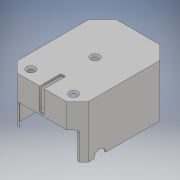
# Autodesk Inventor part: Kozhuh_Lock_Left
Saved by Autodesk Inventor 2017 (Build 210142000, 142)
## iProperties
Part Number: Kozhuh_Lock_Left
Material: Типовые
Document SubType Name: Modeling
Designer: yulia_000
Density: 1 g/cm^3
Appearance: По умолчанию
Author: yulia_000
## iProperties of the stored document Kozhuh_Lock_Right_3DПЕЧАТЬ.ipt
Part Number: Kozhuh_Lock_Right_3DПЕЧАТЬ
Material: Типовые
Document SubType Name: Modeling
Designer: Тетяна
Density: 1 g/cm^3
Appearance: По умолчанию
Author: Тетяна
Autodesk Inventor part; units mm, degrees
ref_plane "YZ Plane" through (0, 0, 0) normal (1, 0, 0) x (0, 1, 0)
ref_plane "XZ Plane" through (0, 0, 0) normal (0, 1, 0) x (-1, 0, 0)
ref_plane "XY Plane" through (0, 0, 0) normal (0, 0, 1) x (1, 0, 0)
sketch "Эскиз1" plane through (0, 0, 0) normal (0, 1, 0) x (-1, 0, 0)
  line L0 (11, 0) -> (47.6, 0)
  line L1 (58.6, -11) -> (58.6, -71.5)
  line L2 (50.1, -80) -> (8.5, -80)
  line L3 (0, -71.5) -> (0, -11)
  line L4 (58.6, -11) -> (47.6, 0)
  line L5 (58.6, -71.5) -> (50.1, -80)
  line L6 (8.5, -80) -> (0, -71.5)
  line L7 (0, -11) -> (11, 0)
  line L8 (59.8, -71.9971) -> (50.5971, -81.2)
  line L9 (50.5971, -81.2) -> (8.0029, -81.2)
  line L10 (8.0029, -81.2) -> (-1.2, -71.9971)
  line L11 (-1.2, -71.9971) -> (-1.2, -10.5029)
  line L12 (-1.2, -10.5029) -> (10.5029, 1.2)
  line L13 (10.5029, 1.2) -> (48.0971, 1.2)
  line L14 (48.0971, 1.2) -> (59.8, -10.5029)
  line L15 (59.8, -10.5029) -> (59.8, -71.9971)
  line L16 (31.3, -63) -> (27.3, -63)
  line L17 (27.3, -63) -> (27.3, -80)
  line L18 (27.3, -80) -> (31.3, -80)
  line L19 (31.3, -80) -> (31.3, -63)
  line L20 (31.3, -63) -> (27.3, -80) construction
  line L21 (27.3, -63) -> (31.3, -80) construction
  point P0 (0, 0)
  point P1 (58.6, -80)
  point P2 (58.6, 0)
  point P3 (0, -80)
  point P4 (29.3, -71.5)
  point P5 (29.3, -80)
  dimension "d8" = 58.6
  dimension "d9" = 80
  dimension "d10" = 11
  dimension "d11" = 11
  dimension "d12" = 8.5
  dimension "d13" = 8.5
  dimension "d14" = 8.5
  dimension "d15" = 8.5
  dimension "d16" = 11
  dimension "d17" = 11
  dimension "d18" = 1.2
  dimension "d51" = 4
  dimension "d52" = 17
  constraints: 44 end point, 8 point on line, 6 parallel, 4 midpoint, 3 perpendicular, 2 horizontal, 7 other
  measures "d8" distance of point (58.6, -80) point (0, -80)
  measures "d9" distance of point (58.6, 0) point (58.6, -80)
  measures "d10" distance of L1.start point (58.6, 0)
  measures "d11" distance of L0.end point (58.6, 0)
  measures "d12" distance of L1.end point (58.6, -80)
  measures "d13" distance of L2.start point (58.6, -80)
  measures "d14" distance of L2.end point (0, -80)
  measures "d15" distance of L3.start point (0, -80)
  measures "d16" distance of L3.end point (0, 0)
  measures "d17" distance of L0.start point (0, 0)
  measures "d18" distance between parallel lines of L1 L15
  measures "d51" distance of L18.end L17.end
  measures "d52" distance of L17.end L16.end
extrude "Выдавливание1" add sketch "Эскиз1" against normal blind 1.5 contours L0 L4 L1 L5 L2 L19 L16 L17 L6 L3 L7 | L17 L16 L19 L2 | L8 L9 L10 L11 L12 L13 L14 L15
extrude "Выдавливание2" add sketch "Эскиз1" along normal blind 43.5
fillet "Сопряжение1" radius 1 8 edges at (-58.6, 0, -41.25) (-54.35, 0, -75.75) (-29.3, 0, -80) (-4.25, 0, -75.75) (0, 0, -41.25) (-5.5, 0, -5.5) (-29.3, 0, 0) (-53.1, 0, -5.5)
extrude "Выдавливание3" add sketch "Эскиз1" along normal blind 18 separate body contours L17 L16 L19 L2
sketch "Эскиз2" plane through (-27.3, 0, -80) normal (0, 0, -1) x (-1, 0, 0)
  line L0 (0, 0) -> (4, 0) projected
  line L1 (4, 0) -> (4, 18) projected
  line L2 (0, 18) -> (4, 18) projected
  line L3 (0, 0) -> (0, 18) projected
  point P0 (-27.3, 0)
extrude "Выдавливание4" add sketch "Эскиз2" along normal blind 17 bodies 2
sketch "Эскиз3" plane through (0, 0, 0) normal (0, -1, 0) x (1, 0, 0)
  line L0 (-27.3, -63) -> (-27.3, -97) projected
  line L1 (-31.3, -63) -> (-27.3, -63) projected
  line L2 (-31.3, -63) -> (-31.3, -97) projected
  line L3 (-27.3, -97) -> (-31.3, -97) projected
  point P0 (0, 0)
extrude "Выдавливание5" add sketch "Эскиз3" along normal blind 18 bodies 2
combine bodies "Комбинировать1" operation type subtract main body 1 bodies to subtract 2
hole "Отверстие4" at (-47.6, -1.5, -72.5) direction (0, 1, 0) diameter 4.2 end through all countersink diameter 7.5 countersink angle 90 bodies 1
hole "Отверстие5" at (-11, -1.5, -72.5) direction (0, 1, 0) diameter 4.2 end through all countersink diameter 7.5 countersink angle 90 bodies 1
hole "Отверстие6" at (-29, -1.5, -36) direction (0, 1, 0) diameter 4.2 end through all countersink diameter 7.5 countersink angle 90 bodies 1
fillet "Сопряжение2" radius 1 16 edges at (-58.3071, 0.2929, -71.3787) (-58.6, 22.25, -71.5) (-49.9787, 0.2929, -79.7071) (-50.1, 22.25, -80) (-8.6213, 0.2929, -79.7071) (-8.5, 22.25, -80) (-0.2929, 0.2929, -71.3787) (0, 22.25, -71.5) (-0.2929, 0.2929, -11.1213) (0, 22.25, -11) (-11.1213, 0.2929, -0.2929) (-11, 22.25, 0) (-47.4787, 0.2929, -0.2929) (-47.6, 22.25, 0) (-58.3071, 0.2929, -11.1213) (-58.6, 22.25, -11)
fillet "Сопряжение3" radius 1 4 edges at (-31.3, -0.75, -63) (-27.3, -0.75, -63) (-27.3, 18, -80.6) (-31.3, 18, -80.6)
sketch "Эскиз4" plane through (-8.0029, 43.5, -81.2) normal (0, 0, -1) x (-1, 0, 0)
  line L0 (42.5941, 0) -> (42.5941, -45) projected
  line L1 (0, 0) -> (42.5941, 0) projected
  line L2 (0, 0) -> (0, -45) projected
  line L3 (42.5941, 0) -> (42.5941, -24)
  line L4 (42.5941, -24) -> (0, -24)
  line L5 (0, -24) -> (0, 0)
  line L6 (0.2042, 0) -> (-7.7101, 0) projected
  line L7 (0, 0) -> (42.5941, 0)
  line L8 (39.8899, 0) -> (50.3042, 0) projected
  point P0 (-8.0029, -43.5)
  dimension "d88" = 24
  constraints: 8 end point, 2 perpendicular, 2 point on line, 1 collinear
  measures "d88" distance of L0.start L3.end
extrude "Выдавливание6" add sketch "Эскиз4" against normal blind 5.5 separate body
sketch "Эскиз5" plane through (-50.5971, 19.5, -81.2) normal (-1, 0, 0) x (0, 0, 1)
  line L0 (0, 0) -> (0, 24) projected
  line L1 (0, 0) -> (5.5, 0) projected
  line L2 (5.5, 24) -> (5.5, 0) projected
  line L3 (0, 24) -> (5.5, 24) projected
  point P0 (81.2, -19.5)
extrude "Выдавливание7" add sketch "Эскиз5" along normal blind 10 bodies 3
sketch "Эскиз6" plane through (-8.0029, 19.5, -81.2) normal (1, 0, 0) x (0, 0, -1)
  line L0 (0, 24) -> (0, 0) projected
  line L1 (0, 24) -> (-5.5, 24) projected
  line L2 (-5.5, 0) -> (-5.5, 24) projected
  line L3 (0, 0) -> (-5.5, 0) projected
  point P0 (-81.2, -19.5)
extrude "Выдавливание8" add sketch "Эскиз6" along normal blind 10 bodies 3
combine bodies "Комбинировать2" operation type subtract main body 1 bodies to subtract 3
fillet "Сопряжение4" radius 2 2 edges at (-55.2485, 19.5, -75.7) (-3.3515, 19.5, -75.7)
ref_plane "РабПлоскость1" through (1.2, 43.5, -71.9971) normal (1, 0, 0) x (0, 0, -1)
sketch "Эскиз9" plane through (1.2, 43.5, -71.9971) normal (1, 0, 0) x (0, 0, -1)
  line L0 (-61.4941, 0) -> (-61.4941, -45) projected
  line L1 (0, -45) -> (-61.4941, -45) projected
  line L2 (0, 0) -> (0, -45) projected
  line L3 (-61.4941, 0) -> (0, 0) projected
  line L4 (-60.5828, 0) -> (-0.9113, 0) projected
  arc A0 (-15, 0) -> (-5, 0) centre (-10, 0) ccw
  point P0 (-71.9971, -43.5)
  dimension "d108" = 10
  dimension "d109" = 5
  dimension "d110" = 5
  constraints: 2 point on circle, 2 point on line, 1 centre point
  measures "d108" distance of A0.end A0.start
  measures "d109" radius of A0
  measures "d110" distance of L2.start A0.end
extrude "Выдавливание11" cut sketch "Эскиз9" against normal blind 10 contours L3 A0 bodies 1
equation "\"d13\" = d12"
